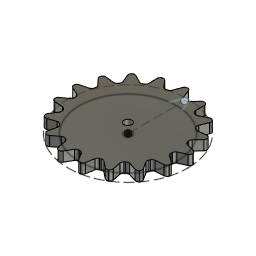
Gear_Template v1 (Autodesk Fusion 360 design; units mm, degrees)
Autodesk Fusion 360 part; units mm, degrees
note: some values were not read from the file. Set by a fixed rule: which sketch regions a step uses.
sketch "Sketch1" plane through (0, 0, 0) normal (0, 0, 1) x (1, 0, 0)
  circle A0 centre (0, 0) radius 1.2
  circle A1 centre (0, 0) radius 15
  circle A2 centre (0, 0) radius 18.5 construction
  line L0 (0, 0) -> (0, 18.5) construction
  line L1 (-0.9168, 17.842) -> (-2, 14.8661)
  line L2 (0.9168, 17.842) -> (2, 14.8661)
  line L3 (-2, 14.8661) -> (2, 14.8661) construction
  line L4 (0.0228, 18.5) -> (-0.0228, 18.5)
  arc A3 (0.0228, 18.5) -> (-0.9168, 17.842) centre (0.0228, 17.5) ccw
  arc A4 (0.9168, 17.842) -> (-0.0228, 18.5) centre (-0.0228, 17.5) ccw
  dimension "d4" = 2.4
  dimension "d5" = 30
  dimension "d6" = 37
  dimension "d12" = 70
  dimension "d14" = 4
  dimension "d24" = 1
  constraint coincident A0.centre A1.centre
  constraint concentric A0 A2
  constraint coincident A2 L0.end
  constraint vertical L0
  constraint coincident A1 L1.end
  constraint coincident A1 L2.end
  constraint symmetric L0 L1 L2
  constraint tangent L4 A3
  constraint tangent L1 A3
  constraint symmetric L0 L4.start L4.end
  constraint symmetric L0 L1.start L2.start
  constraint symmetric L0 A3 A4
  constraint coincident A2 L4.start
  measures "d4" diameter of A0
  measures "d5" diameter of A1
  measures "d6" diameter of A2
  measures "d12" angle of L1 L3
  measures "d14" distance of L1.end L2.end
  measures "d24" radius of A3
extrude "Extrude1" add sketch "Sketch1" along normal blind 3 contours A1
extrude "Extrude2" add sketch "Sketch1" along normal blind 3 contours A1 L1 L2 L4 A3 A4
fillet "Fillet1" radius 1 2 edges at (-2, 14.8661, 1.5) (2, 14.8661, 1.5)
pattern_circular "C-Pattern2" count 17 over 360 about axis through (0, 0, 3) along (0, 0, 1) of "Extrude2", "Fillet1"
equation "Rod_Diameter = 2.4 mm"
equation "Inner_Diameter = 30 mm"
equation "Gear_Diameter = Inner_Diameter + Tooth_Size"
equation "d4 = Rod_Diameter"
equation "d5 = Inner_Diameter"
equation "d6 = Gear_Diameter"
equation "Tooth_Angle = 70 deg"
equation "d12 = Tooth_Angle"
equation "Tooth_Base = 4 mm"
equation "d14 = Tooth_Base"
equation "d16 = Gear_Thickness"
equation "d18 = Gear_Thickness"
equation "Tooth_Number = 17"
equation "Gear_Thickness = 3 mm"
equation "d24 = Fillet_Radius"
equation "Fillet_Radius = 1 mm"
equation "d28 = Fillet_Radius"
equation "d29 = Tooth_Number"
equation "Tooth_Size = 7 mm"
